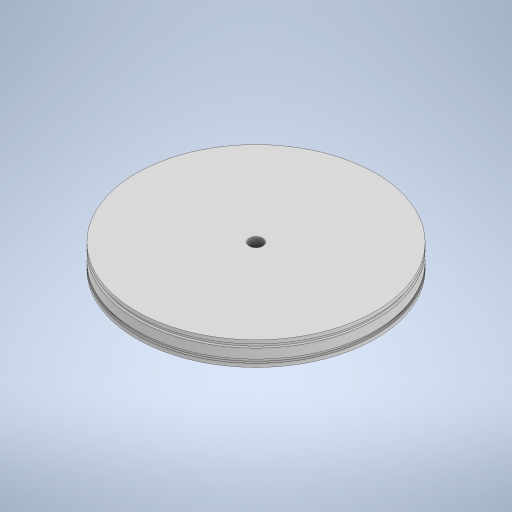
# Autodesk Inventor part: Piston Head
Saved by Autodesk Inventor 2023 (Build 270158030, 158C)
## iProperties
Created: 2022-09-17
Part Number: Piston Head
Material: Generic
Document SubType Name: Modeling
Designer: cjj5381
Density: 1 g/cm^3
Appearance: Default
Author: cjj5381
Autodesk Inventor part; units mm, degrees
ref_plane "YZ Plane" through (0, 0, 0) normal (1, 0, 0) x (0, 1, 0)
ref_plane "XZ Plane" through (0, 0, 0) normal (0, 1, 0) x (-1, 0, 0)
ref_plane "XY Plane" through (0, 0, 0) normal (0, 0, 1) x (1, 0, 0)
sketch "Sketch1" plane through (0, 0, 0) normal (0, 1, 0) x (-1, 0, 0)
  circle A0 centre (0, 0) radius 63.5
  dimension "d0" = 127
  constraints: 1 centre point, 1 coincident
  measures "d0" diameter of A0
extrude "Extrusion1" add sketch "Sketch1" along normal blind 12.7
sketch "Sketch2" plane through (0, 12.7, 0) normal (0, 1, 0) x (1, 0, 0)
  point P0 (0, 0)
  point P1 (26.4475, 5.8254)
hole "Hole1" at (0, 12.7, 0) direction (0, -1, 0) diameter 7.1374 end through all clearance for "Hex Head Bolt" size "1/4" standard "Ansi Unified Screw Threads"
sketch "Sketch3" plane through (0, 0, 0) normal (0, -1, 0) x (1, 0, 0)
  circle A0 centre (0, 0) radius 3.5687 projected
  line L0 (6.4231, 0) -> (3.2116, -5.5626)
  line L1 (3.2116, -5.5626) -> (-3.2116, -5.5626)
  line L2 (-3.2116, -5.5626) -> (-6.4231, 0)
  line L3 (-6.4231, 0) -> (-3.2116, 5.5626)
  line L4 (-3.2116, 5.5626) -> (3.2116, 5.5626)
  line L5 (3.2116, 5.5626) -> (6.4231, 0)
  dimension "d10" = 11.1252
  constraints: 12 end point, 1 coincident, 13 other
  measures "d10" distance between parallel lines of L1 L4
extrude "Extrusion2" cut sketch "Sketch3" against normal blind 4.3688 contours A0 | L0 L1 L2 L3 L4 L5
chamfer "Chamfer1" distance 0.508 angle 45 6 edges at (4.8174, 0, 2.7813) (0, 0, 5.5626) (-4.8174, 0, 2.7813) (-4.8174, 0, -2.7813) (0, 0, -5.5626) (4.8174, 0, -2.7813)
sketch "Sketch4" plane through (0, 0, 0) normal (0, 0, 1) x (1, 0, 0)
  line L0 (-63.5, 0) -> (-63.5, 12.7) projected
  line L1 (-63.5, 3.81) -> (-62.23, 3.81)
  line L2 (-62.23, 3.81) -> (-62.23, 1.905)
  line L3 (-62.23, 1.905) -> (-63.5, 1.905)
  line L4 (-63.5, 1.905) -> (-63.5, 3.81)
  line L5 (-63.5, 10.795) -> (-62.23, 10.795)
  line L6 (-62.23, 10.795) -> (-62.23, 8.89)
  line L7 (-62.23, 8.89) -> (-63.5, 8.89)
  line L8 (-63.5, 8.89) -> (-63.5, 10.795)
  line L9 (-63.5, 6.35) -> (-70.565, 6.35)
  line L10 (0, 0) -> (0, 18.3077)
  dimension "d16" = 1.27
  dimension "d17" = 1.905
  dimension "d18" = 5.08
  constraints: 20 end point, 4 parallel, 3 horizontal, 3 point on line, 2 perpendicular, 1 collinear, 1 midpoint, 1 vertical, 1 other
  measures "d16" distance of L2.end L3.end
  measures "d17" distance of L1.end L2.end
  measures "d18" distance between parallel lines of L7 L1
revolve "Revolution1" cut sketch "Sketch4" angle 360 about axis through (0, 0, 0) along (0, 1, 0)
body "Solid1"
